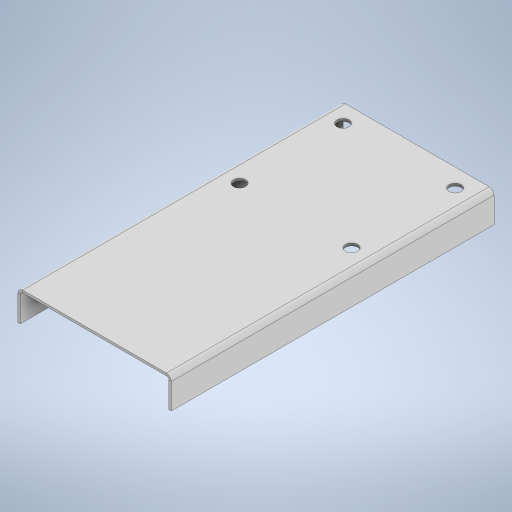
# Autodesk Inventor part: Крепление
Saved by Autodesk Inventor 2024.2 (Build 282272000, 272)
## iProperties
Created: 2024-04-09
Part Number: Крепление
Material: Generic
Document SubType Name: Sheet Metal
Designer: pokla
Density: 1 g/cm^3
Sheet Metal Rule: Default_mm
Appearance: Default
Flat Pattern Width: 16.9048 cm
Flat Pattern Length: 26.5 cm
Flat Pattern Area: 447.977 cm^2
Sheet Metal Width: 169,048 mm
Sheet Metal Length: 265,000 mm
Sheet Metal Area: 44797,664 mm^2
Author: pokla
Autodesk Inventor part; units mm, degrees
ref_plane "YZ Plane" through (0, 0, 0) normal (1, 0, 0) x (0, 1, 0)
ref_plane "XZ Plane" through (0, 0, 0) normal (0, 1, 0) x (-1, 0, 0)
ref_plane "XY Plane" through (0, 0, 0) normal (0, 0, 1) x (1, 0, 0)
sketch "Sketch4" plane through (0, 0, 0) normal (0, 1, 0) x (-1, 0, 0)
  line L0 (63, -132.5) -> (-63, -132.5)
  line L1 (-63, -132.5) -> (-63, 132.5)
  line L2 (-63, 132.5) -> (63, 132.5)
  line L3 (63, 132.5) -> (63, -132.5)
  line L4 (63, -132.5) -> (-63, 132.5) construction
  point P0 (0, 0)
  point P1 (0, 0)
  dimension "d24" = 126
  dimension "d25" = 265
  measures "d24" distance of L1.end L2.end
  measures "d25" distance of L0.end L1.end
extrude "Plate4" add sketch "Sketch4" along normal mid plane 2
sketch "Sketch7" plane through (0, -1, 0) normal (0, -1, 0) x (1, 0, 0)
  circle A0 centre (46, -117.5) radius 5
  line L0 (63, 132.5) -> (63, -132.5) projected
  line L1 (63, -132.5) -> (-63, -132.5) projected
  line L2 (0, -74.3103) -> (0, 74.3103) construction
  line L3 (114.9724, 0) -> (-114.9724, 0) construction
  circle A1 centre (-46, -117.5) radius 5
  circle A2 centre (46, -32.5) radius 5
  circle A3 centre (-46, -32.5) radius 5
  point P0 (0, 0)
  point P1 (0, 0)
  dimension "d41" = 10
  dimension "d42" = 17
  dimension "d43" = 15
  dimension "d46" = 85
  constraints: 4 centre point, 4 end point, 2 equal radius, 2 midpoint, 2 vertical alignment, 1 coincident, 1 horizontal, 1 horizontal alignment, 1 symmetric about line, 1 vertical, 1 other
  measures "d41" diameter of A0
  measures "d42" distance from line of L0 A0.centre
  measures "d43" distance from line of L1 A0.centre
  measures "d46" distance of A1.centre A3.centre
extrude "Extrusion2" cut sketch "Sketch7" against normal up to surface (2 mm away)
sketch "Sketch8" plane through (61, 1, 132.5) normal (1, 0, 0) x (0, 1, 0)
  line L0 (0, -265) -> (0, 0)
  line L1 (0, 0) -> (-25, 0)
  line L2 (-25, 0) -> (-25, -265)
  line L3 (-25, -265) -> (0, -265)
  constraints: 6 end point, 1 horizontal, 1 perpendicular, 1 vertical
edge flange "Flange4" height 25 angle 90 thickness 2 bend radius 2 thickness toward (1, 0, 0) relief tear relief width 2 relief depth 1 corner gap 2 corner form 0 edges at (63, -1, 0) (-63, -1, 0) wall of the first edge with corners at (61, 1, -132.5) (61, 1, 132.5) (61, -24, 132.5) (61, -24, -132.5)
bend "Bend4"
corner "Corner4"
equation "\"d26\" = Thickness"
equation "\"d47\" = BendReliefWidth"
equation "\"d48\" = BendReliefDepth"
equation "\"d49\" = MinimumRemnant"
equation "\"d50\" = TransitionRadius"
equation "\"d53\" = BendRadius"
equation "\"d54\" = CornerReliefSize"
equation "\"d55\" = GapSize"
equation "\"d56\" = JacobiRadiusSize"
equation "\"BendRadius\" = Thickness"
equation "\"BendReliefWidth\" = Thickness"
equation "\"BendReliefDepth\" = 0.5 * Thickness"
equation "\"CornerReliefSize\" = 4 * Thickness"
equation "\"MinimumRemnant\" = 2 * Thickness"
equation "\"TransitionRadius\" = BendRadius"
equation "\"JacobiRadiusSize\" = BendRadius"
equation "\"GapSize\" = Thickness"
equation "\"Thickness\" = 2"
body "Solid2"
